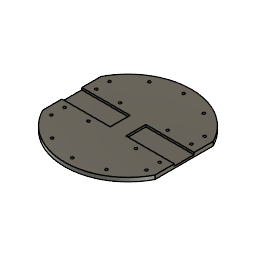
Chasis (Autodesk Fusion 360 design; units mm, degrees)
part number: 2026-04-02-12-40-59-312
Autodesk Fusion 360 part; units mm, degrees
sketch "Sketch1" plane through (0, 0, 0) normal (0, 0, 1) x (-1, 0, 0)
  line L0 (-80, 0) -> (80, 0) construction
  line L1 (-71, -12.5) -> (-10, -12.5)
  line L2 (-10, -12.5) -> (-10, 12.5)
  line L3 (-10, 12.5) -> (-71, 12.5)
  line L4 (-71, 12.5) -> (-71, -12.5)
  line L5 (-71, -36.8646) -> (-71, 36.8646)
  line L6 (0, -80) -> (0, 80) construction
  line L7 (10, -12.5) -> (10, 12.5)
  line L8 (10, 12.5) -> (71, 12.5)
  line L9 (71, -12.5) -> (10, -12.5)
  line L10 (71, 12.5) -> (71, -12.5)
  line L11 (71, -36.8646) -> (71, 36.8646)
  arc A0 (71, 36.8646) -> (-71, 36.8646) centre (0, 0) ccw
  arc A1 (-71, -36.8646) -> (71, -36.8646) centre (0, 0) ccw
  dimension "d6" = 160
  dimension "d7" = 61
  dimension "d8" = 25
  dimension "d9" = 10
  dimension "d10" = 71
  constraint coincident A0.centre A1.centre
  constraint horizontal L0
  constraint horizontal L1
  constraint vertical L2
  constraint horizontal L3
  constraint vertical L4
  constraint symmetric L0 L1 L3
  constraint perpendicular L3 L5
  constraint coincident L6.start A1
  constraint coincident L6.end A0
  constraint vertical L6
  constraint symmetric L1.start L6 L9.start
  constraint symmetric L1.end L6 L7.start
  constraint symmetric L2.end L6 L7.end
  constraint symmetric L3.end L6 L8.end
  constraint symmetric L5.start L6 L11.start
  constraint symmetric L5.end L6 L11.end
  constraint concentric A0 A1
  measures "d6" diameter of A0
  measures "d7" distance of L1.start L1.end
  measures "d8" distance of L1.start L3.end
  measures "d9" distance of A0.centre L2
  measures "d10" distance of A0.centre L5
extrude "Extrude1" add sketch "Sketch1" along normal blind 5 contours L1 L2 L3 L5 L7 L8 L9 L11 A0 A1
sketch "Sketch2" plane through (0, 0, 5) normal (0, 0, 1) x (-1, 0, 0)
  line L0 (-71, -12.5) -> (-71, -36.8646)
  arc A0 (-71, -36.8646) -> (71, -36.8646) centre (0, 0) ccw
  line L1 (71, -36.8646) -> (71, -12.5)
  line L2 (71, -12.5) -> (10, -12.5)
  line L3 (10, -12.5) -> (10, 12.5)
  line L4 (10, 12.5) -> (71, 12.5)
  line L5 (71, 12.5) -> (71, 36.8646)
  arc A1 (71, 36.8646) -> (-71, 36.8646) centre (0, 0) ccw
  line L6 (-71, 36.8646) -> (-71, 12.5)
  line L7 (-71, 12.5) -> (-10, 12.5)
  line L8 (-10, 12.5) -> (-10, -12.5)
  line L9 (-10, -12.5) -> (-71, -12.5)
  line L10 (-71, 12.5) -> (-10, 12.5)
  line L11 (-10, 12.5) -> (-10, -12.5)
  line L12 (-10, -12.5) -> (-71, -12.5)
  line L13 (10, 12.5) -> (71, 12.5)
  line L14 (10, -12.5) -> (10, 12.5)
  line L15 (71, -12.5) -> (10, -12.5)
  line L16 (-71, -12.5) -> (-71, 12.5)
  line L17 (71, -12.5) -> (71, 12.5)
  constraint coincident L0.start L9.end
  constraint coincident L6.end L7.start
  constraint coincident L1.end L2.start
  constraint coincident L4.end L5.start
extrude "Extrude2" add sketch "Sketch2" against normal blind 2.5 contours L7 L8 L9 L10 L11 L12 L16 | L2 L3 L4 L13 L14 L15 L17
move_body "Move1" bodies 1 to x (1, 0, 0) y (0, -1, 0) z (0, 0, -1) at (0, 0, 0)
move_body "Move2" bodies 1 to x (1, 0, 0) y (0, 1, 0) z (0, 0, 1) at (0, 0, 5)
sketch "Sketch3" plane through (0, 0, 5) normal (0, 0, 1) x (-1, 0, 0)
  line L0 (-71, 36.8646) -> (-71, 12.5)
  line L1 (-71, 12.5) -> (-10, 12.5)
  line L2 (-10, 12.5) -> (-10, -12.5)
  line L3 (-10, -12.5) -> (-71, -12.5)
  line L4 (-71, -12.5) -> (-71, -36.8646)
  arc A0 (-71, -36.8646) -> (71, -36.8646) centre (0, 0) ccw
  line L5 (71, -36.8646) -> (71, -12.5)
  line L6 (71, -12.5) -> (10, -12.5)
  line L7 (10, -12.5) -> (10, 12.5)
  line L8 (10, 12.5) -> (71, 12.5)
  line L9 (71, 12.5) -> (71, 36.8646)
  arc A1 (71, 36.8646) -> (-71, 36.8646) centre (0, 0) ccw
  line L10 (-70, 0) -> (70, 0) construction
  line L11 (0, 80) -> (0, -80) construction
  point P0 (-60.0095, 36.8646)
  point P1 (-34.3452, 61.4862)
  point P2 (0.0774, 70.4282)
  point P3 (34.4802, 61.4105)
  point P4 (60.0904, 36.7327)
  point P5 (-60.0095, -36.8646)
  point P6 (-34.3452, -61.4862)
  point P7 (0.0774, -70.4282)
  point P8 (34.4802, -61.4105)
  point P9 (60.0904, -36.7327)
  point P10 (-60, 20)
  point P11 (-30, 20)
  point P12 (-60, -20)
  point P13 (-30, -20)
  point P14 (60, 20)
  point P15 (30, 20)
  point P16 (60, -20)
  point P17 (30, -20)
  dimension "d20" = -117
  constraint perpendicular L7 L10
  constraint symmetric P0 L10 P5
  constraint symmetric P1 L10 P6
  constraint symmetric P2 L10 P7
  constraint symmetric P3 L10 P8
  constraint symmetric P4 L10 P9
  constraint midpoint A1 L11.start
  constraint midpoint A0 L11.end
  constraint symmetric L10 P10 P12
  constraint symmetric L10 P11 P13
  constraint symmetric P10 L11 P14
  constraint symmetric P11 L11 P15
  constraint symmetric L11 P12 P16
  constraint symmetric L11 P13 P17
hole "Hole1" at (60, -20, 5) at (60.0095, -36.8646, 5) at (34.3452, -61.4862, 5) at (-0.0774, -70.4282, 5) at (-34.4802, -61.4105, 5) at (-30, -20, 5) at (-60, -20, 5) at (-60.0904, -36.7327, 5) at (-30, 20, 5) at (-60, 20, 5) at (-60.0904, 36.7327, 5) at (-34.4802, 61.4105, 5) at (-0.0774, 70.4282, 5) at (30, 20, 5) at (60, 20, 5) at (60.0095, 36.8646, 5) at (34.3452, 61.4862, 5) at (30, -20, 5) direction (0, 0, -1) diameter 3.2 end through all
equation "chasis_diameter = 160 mm"
equation "main_layer_thickness = 30 mm"
equation "motor_L = 21 mm"
equation "total_motor_body_length = 61 mm"
equation "standoff_height = 50 mm"
equation "d6 = chasis_diameter"
